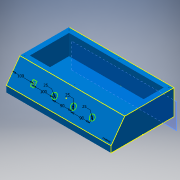
# Autodesk Inventor part: 240710_part2
Saved by Autodesk Inventor 2016 (Build 200138000, 138)
## iProperties
Created: 2024-07-10
Part Number: 240710_part2
Material: 일반
Document SubType Name: Modeling
Designer: pc
Density: 1 g/cm^3
Appearance: 기본값(1)
Author: pc
Autodesk Inventor part; units mm, degrees
ref_plane "YZ Plane" through (0, 0, 0) normal (1, 0, 0) x (0, 1, 0)
ref_plane "XZ Plane" through (0, 0, 0) normal (0, 1, 0) x (-1, 0, 0)
ref_plane "XY Plane" through (0, 0, 0) normal (0, 0, 1) x (1, 0, 0)
sketch "스케치1" plane through (0, 0, 0) normal (0, 0, 1) x (1, 0, 0)
  line L0 (250, -150) -> (-250, -150)
  line L1 (-250, -150) -> (-250, 150)
  line L2 (-250, 150) -> (250, 150)
  line L3 (250, 150) -> (250, -150)
  line L4 (250, -150) -> (-250, 150) construction
  line L5 (-250, -150) -> (250, 150) construction
  point P0 (0, 0)
  dimension "d0" = 500
  dimension "d1" = 300
  constraints: 12 end point, 2 midpoint, 2 parallel, 1 horizontal, 1 perpendicular
  measures "d0" distance of L1.end L2.end
  measures "d1" distance of L0.end L1.end
extrude "돌출1" add sketch "스케치1" along normal blind 120
sketch "스케치2" plane through (250, -150, 0) normal (1, 0, 0) x (0, 0, -1)
  line L0 (-120, 0) -> (-120, 300) projected
  line L1 (0, 0) -> (-120, 0) projected
  line L2 (-30, 0) -> (-120, 65)
  line L3 (-30, 0) -> (-30, -74.841)
  line L4 (-30, -74.841) -> (-182.9501, -91.3391)
  line L5 (-182.9501, -91.3391) -> (-221.4457, -10.4199)
  line L6 (-221.4457, -10.4199) -> (-120, 65)
  point P0 (0, 150)
  dimension "d4" = 65
  dimension "d5" = 30
  constraints: 10 end point, 2 point on line, 1 vertical
  measures "d4" distance of L2.end L0.start
  measures "d5" distance of L1.start L2.start
extrude "돌출2" cut sketch "스케치2" against normal through all contours L0 L2 L1
sketch "스케치3" plane through (0, 0, 120) normal (0, 0, 1) x (1, 0, 0)
  line L0 (-250, -85) -> (250, -85) projected
  line L1 (250, -85) -> (250, 150) projected
  line L2 (250, 150) -> (-250, 150) projected
  line L3 (-250, 150) -> (-250, -85) projected
  line L4 (-226, -61) -> (226, -61)
  line L5 (226, -61) -> (226, 126)
  line L6 (226, 126) -> (-226, 126)
  line L7 (-226, 126) -> (-226, -61)
  point P0 (0, 0)
  dimension "d8" = 24
  dimension "d9" = 24
  dimension "d10" = 24
  dimension "d11" = 24
  constraints: 8 end point, 2 parallel, 1 horizontal, 1 perpendicular
  measures "d8" distance between parallel lines of L3 L7
  measures "d9" distance between parallel lines of L2 L6
  measures "d10" distance between parallel lines of L0 L4
  measures "d11" distance between parallel lines of L1 L5
extrude "돌출3" cut sketch "스케치3" against normal blind 10 contours L7 L6 L5 L4
shell "쉘1" thickness 1.2 removed faces 5 at (-226, 63.6667, 116.6667) at (-75.3333, -61, 116.6667) at (226, 1.3333, 116.6667) at (75.3333, 126, 116.6667) at (75.3333, 1.3333, 110)
sketch "스케치4" plane through (0, 0, 120) normal (0, 0, 1) x (1, 0, 0)
  line L0 (-250, -85) -> (250, -85) projected
  line L1 (250, -85) -> (250, 150) projected
  line L2 (250, 150) -> (-250, 150) projected
  line L3 (-250, 150) -> (-250, -85) projected
  line L4 (-238, -73) -> (238, -73)
  line L5 (238, -73) -> (238, 138)
  line L6 (238, 138) -> (-238, 138)
  line L7 (-238, 138) -> (-238, -73)
  line L8 (-238, 32.5) -> (250, 32.5)
  line L9 (0, -73) -> (0, 138)
  point P0 (0, 0)
  dimension "d15" = 12
  dimension "d16" = 12
  dimension "d17" = 12
  dimension "d18" = 12
  constraints: 12 end point, 6 coincident, 4 midpoint, 2 parallel, 1 horizontal, 1 perpendicular
  measures "d15" distance between parallel lines of L0 L4
  measures "d16" distance between parallel lines of L3 L7
  measures "d17" distance between parallel lines of L2 L6
  measures "d18" distance between parallel lines of L1 L5
hole "구멍1" at (-238, -73, 120) at (-238, 138, 120) at (238, -73, 120) at (238, 138, 120) at (0, -73, 120) at (0, 138, 120) direction (0, 0, -1) diameter 4.134 depth 14.2 tip angle 118 thread size "M5x0.8" class "6H" standard "ISO Metric profile"
sketch "스케치5" plane through (-250, -150, 30) normal (0, -0.8107, 0.5855) x (1, 0, 0)
  line L0 (0, 0) -> (0, 111.018) projected
  circle A0 centre (200, 51.355) radius 12.5
  circle A1 centre (290, 51.355) radius 12.5
  circle A2 centre (380, 51.355) radius 12.5
  line L1 (109.038, 38.855) -> (90.962, 38.855)
  line L2 (90.962, 38.855) -> (90.962, 63.855)
  line L3 (90.962, 63.855) -> (109.038, 63.855)
  line L4 (109.038, 63.855) -> (109.038, 38.855)
  line L5 (109.038, 38.855) -> (90.962, 63.855) construction
  line L6 (90.962, 38.855) -> (109.038, 63.855) construction
  line L7 (455.4394, 12.1665) -> (493.5306, 12.1665) construction
  line L8 (493.5306, 12.1665) -> (493.5306, 2.974) construction
  line L9 (493.5306, 2.974) -> (455.4394, 2.974) construction
  line L10 (455.4394, 2.974) -> (455.4394, 12.1665) construction
  point P0 (250, 63.5032)
  point P1 (100, 51.355)
  dimension "d26" = 25
  dimension "d27" = 25
  dimension "d28" = 25
  dimension "d29" = 100
  dimension "d30" = 100
  dimension "d31" = 90
  dimension "d32" = 90
  constraints: 12 end point, 3 centre point, 2 midpoint, 2 parallel, 1 horizontal, 1 perpendicular, 2 other
  measures "d26" diameter of A0
  measures "d27" diameter of A1
  measures "d28" diameter of A2
  measures "d29" distance from line of L0 point (100, 51.355)
  measures "d30" distance of A0.centre point (100, 51.355)
  measures "d31" distance of A0.centre A1.centre
  measures "d32" distance of A2.centre A1.centre
sketch "스케치6" plane through (250, -150, 0) normal (1, 0, 0) x (0, 0, -1)
  line L0 (-120, 65) -> (-30, 0) projected
  line L1 (0, 0) -> (-30, 0) projected
  line L2 (0, 300) -> (0, 0) projected
  line L3 (0, 300) -> (-120, 300) projected
  line L4 (-120, 65) -> (-120, 300) projected
  point P0 (0, 150)
sketch "스케치7" plane through (250, -150, 0) normal (1, 0, 0) x (0, 0, -1)
  line L0 (-120, 65) -> (-30, 0) projected
  line L1 (0, 0) -> (-30, 0) projected
  line L2 (0, 300) -> (0, 0) projected
  line L3 (0, 300) -> (-120, 300) projected
  line L4 (-120, 65) -> (-120, 300) projected
  point P0 (0, 150)
sketch "스케치8" plane through (-250, 150, 0) normal (0, 1, 0) x (1, 0, 0)
  line L0 (0, 0) -> (500, 0) projected
  line L1 (0, 0) -> (0, -120) projected
  line L2 (500, -120) -> (0, -120) projected
  line L3 (500, 0) -> (500, -120) projected
  point P0 (250, 0)
sketch "스케치9" plane through (-250, 150, 0) normal (0, 1, 0) x (1, 0, 0)
  line L0 (446.8349, -55.3209) -> (487.5108, -55.3209) construction
  line L1 (451.514, -50.6418) -> (482.8317, -50.6418)
  line L2 (482.8317, -60) -> (451.514, -60)
  arc A0 (451.514, -50.6418) -> (451.514, -60) centre (451.514, -55.3209) ccw
  arc A1 (482.8317, -60) -> (482.8317, -50.6418) centre (482.8317, -55.3209) ccw
  line L3 (515.6985, -42.8327) -> (515.6985, 0) construction
  line L4 (432.8317, -60) -> (401.514, -60)
  line L5 (401.514, -50.6418) -> (432.8317, -50.6418)
  arc A2 (401.514, -50.6418) -> (401.514, -60) centre (401.514, -55.3209) ccw
  arc A3 (432.8317, -60) -> (432.8317, -50.6418) centre (432.8317, -55.3209) ccw
  line L6 (382.8317, -60) -> (351.514, -60)
  line L7 (351.514, -50.6418) -> (382.8317, -50.6418)
  arc A4 (351.514, -50.6418) -> (351.514, -60) centre (351.514, -55.3209) ccw
  arc A5 (382.8317, -60) -> (382.8317, -50.6418) centre (382.8317, -55.3209) ccw
  line L8 (332.8317, -60) -> (301.514, -60)
  line L9 (301.514, -50.6418) -> (332.8317, -50.6418)
  arc A6 (301.514, -50.6418) -> (301.514, -60) centre (301.514, -55.3209) ccw
  arc A7 (332.8317, -60) -> (332.8317, -50.6418) centre (332.8317, -55.3209) ccw
  line L10 (282.8317, -60) -> (251.514, -60)
  line L11 (251.514, -50.6418) -> (282.8317, -50.6418)
  arc A8 (251.514, -50.6418) -> (251.514, -60) centre (251.514, -55.3209) ccw
  arc A9 (282.8317, -60) -> (282.8317, -50.6418) centre (282.8317, -55.3209) ccw
  line L12 (232.8317, -60) -> (201.514, -60)
  line L13 (201.514, -50.6418) -> (232.8317, -50.6418)
  arc A10 (201.514, -50.6418) -> (201.514, -60) centre (201.514, -55.3209) ccw
  arc A11 (232.8317, -60) -> (232.8317, -50.6418) centre (232.8317, -55.3209) ccw
  line L14 (182.8317, -60) -> (151.514, -60)
  line L15 (151.514, -50.6418) -> (182.8317, -50.6418)
  arc A12 (151.514, -50.6418) -> (151.514, -60) centre (151.514, -55.3209) ccw
  arc A13 (182.8317, -60) -> (182.8317, -50.6418) centre (182.8317, -55.3209) ccw
  line L16 (132.8317, -60) -> (101.514, -60)
  line L17 (101.514, -50.6418) -> (132.8317, -50.6418)
  arc A14 (101.514, -50.6418) -> (101.514, -60) centre (101.514, -55.3209) ccw
  arc A15 (132.8317, -60) -> (132.8317, -50.6418) centre (132.8317, -55.3209) ccw
  line L18 (82.8317, -60) -> (51.514, -60)
  line L19 (51.514, -50.6418) -> (82.8317, -50.6418)
  arc A16 (51.514, -50.6418) -> (51.514, -60) centre (51.514, -55.3209) ccw
  arc A17 (82.8317, -60) -> (82.8317, -50.6418) centre (82.8317, -55.3209) ccw
  line L20 (482.8317, -45) -> (451.514, -45)
  line L21 (451.514, -35.6418) -> (482.8317, -35.6418)
  arc A18 (451.514, -35.6418) -> (451.514, -45) centre (451.514, -40.3209) ccw
  arc A19 (482.8317, -45) -> (482.8317, -35.6418) centre (482.8317, -40.3209) ccw
  line L22 (432.8317, -45) -> (401.514, -45)
  line L23 (401.514, -35.6418) -> (432.8317, -35.6418)
  arc A20 (401.514, -35.6418) -> (401.514, -45) centre (401.514, -40.3209) ccw
  arc A21 (432.8317, -45) -> (432.8317, -35.6418) centre (432.8317, -40.3209) ccw
  line L24 (382.8317, -45) -> (351.514, -45)
  line L25 (351.514, -35.6418) -> (382.8317, -35.6418)
  arc A22 (351.514, -35.6418) -> (351.514, -45) centre (351.514, -40.3209) ccw
  arc A23 (382.8317, -45) -> (382.8317, -35.6418) centre (382.8317, -40.3209) ccw
  line L26 (332.8317, -45) -> (301.514, -45)
  line L27 (301.514, -35.6418) -> (332.8317, -35.6418)
  arc A24 (301.514, -35.6418) -> (301.514, -45) centre (301.514, -40.3209) ccw
  arc A25 (332.8317, -45) -> (332.8317, -35.6418) centre (332.8317, -40.3209) ccw
  line L28 (282.8317, -45) -> (251.514, -45)
  line L29 (251.514, -35.6418) -> (282.8317, -35.6418)
  arc A26 (251.514, -35.6418) -> (251.514, -45) centre (251.514, -40.3209) ccw
  arc A27 (282.8317, -45) -> (282.8317, -35.6418) centre (282.8317, -40.3209) ccw
  line L30 (232.8317, -45) -> (201.514, -45)
  line L31 (201.514, -35.6418) -> (232.8317, -35.6418)
  arc A28 (201.514, -35.6418) -> (201.514, -45) centre (201.514, -40.3209) ccw
  arc A29 (232.8317, -45) -> (232.8317, -35.6418) centre (232.8317, -40.3209) ccw
  line L32 (182.8317, -45) -> (151.514, -45)
  line L33 (151.514, -35.6418) -> (182.8317, -35.6418)
  arc A30 (151.514, -35.6418) -> (151.514, -45) centre (151.514, -40.3209) ccw
  arc A31 (182.8317, -45) -> (182.8317, -35.6418) centre (182.8317, -40.3209) ccw
  line L34 (132.8317, -45) -> (101.514, -45)
  line L35 (101.514, -35.6418) -> (132.8317, -35.6418)
  arc A32 (101.514, -35.6418) -> (101.514, -45) centre (101.514, -40.3209) ccw
  arc A33 (132.8317, -45) -> (132.8317, -35.6418) centre (132.8317, -40.3209) ccw
  line L36 (82.8317, -45) -> (51.514, -45)
  line L37 (51.514, -35.6418) -> (82.8317, -35.6418)
  arc A34 (51.514, -35.6418) -> (51.514, -45) centre (51.514, -40.3209) ccw
  arc A35 (82.8317, -45) -> (82.8317, -35.6418) centre (82.8317, -40.3209) ccw
  line L38 (482.8317, -30) -> (451.514, -30)
  line L39 (451.514, -20.6418) -> (482.8317, -20.6418)
  arc A36 (451.514, -20.6418) -> (451.514, -30) centre (451.514, -25.3209) ccw
  arc A37 (482.8317, -30) -> (482.8317, -20.6418) centre (482.8317, -25.3209) ccw
  line L40 (432.8317, -30) -> (401.514, -30)
  line L41 (401.514, -20.6418) -> (432.8317, -20.6418)
  arc A38 (401.514, -20.6418) -> (401.514, -30) centre (401.514, -25.3209) ccw
  arc A39 (432.8317, -30) -> (432.8317, -20.6418) centre (432.8317, -25.3209) ccw
  line L42 (382.8317, -30) -> (351.514, -30)
  line L43 (351.514, -20.6418) -> (382.8317, -20.6418)
  arc A40 (351.514, -20.6418) -> (351.514, -30) centre (351.514, -25.3209) ccw
  arc A41 (382.8317, -30) -> (382.8317, -20.6418) centre (382.8317, -25.3209) ccw
  line L44 (332.8317, -30) -> (301.514, -30)
  line L45 (301.514, -20.6418) -> (332.8317, -20.6418)
  arc A42 (301.514, -20.6418) -> (301.514, -30) centre (301.514, -25.3209) ccw
  arc A43 (332.8317, -30) -> (332.8317, -20.6418) centre (332.8317, -25.3209) ccw
  line L46 (282.8317, -30) -> (251.514, -30)
  line L47 (251.514, -20.6418) -> (282.8317, -20.6418)
  arc A44 (251.514, -20.6418) -> (251.514, -30) centre (251.514, -25.3209) ccw
  arc A45 (282.8317, -30) -> (282.8317, -20.6418) centre (282.8317, -25.3209) ccw
  line L48 (232.8317, -30) -> (201.514, -30)
  line L49 (201.514, -20.6418) -> (232.8317, -20.6418)
  arc A46 (201.514, -20.6418) -> (201.514, -30) centre (201.514, -25.3209) ccw
  arc A47 (232.8317, -30) -> (232.8317, -20.6418) centre (232.8317, -25.3209) ccw
  line L50 (182.8317, -30) -> (151.514, -30)
  line L51 (151.514, -20.6418) -> (182.8317, -20.6418)
  arc A48 (151.514, -20.6418) -> (151.514, -30) centre (151.514, -25.3209) ccw
  arc A49 (182.8317, -30) -> (182.8317, -20.6418) centre (182.8317, -25.3209) ccw
  line L52 (132.8317, -30) -> (101.514, -30)
  line L53 (101.514, -20.6418) -> (132.8317, -20.6418)
  arc A50 (101.514, -20.6418) -> (101.514, -30) centre (101.514, -25.3209) ccw
  arc A51 (132.8317, -30) -> (132.8317, -20.6418) centre (132.8317, -25.3209) ccw
  line L54 (82.8317, -30) -> (51.514, -30)
  line L55 (51.514, -20.6418) -> (82.8317, -20.6418)
  arc A52 (51.514, -20.6418) -> (51.514, -30) centre (51.514, -25.3209) ccw
  arc A53 (82.8317, -30) -> (82.8317, -20.6418) centre (82.8317, -25.3209) ccw
  point P0 (250, 0)
  point P1 (467.1729, -55.3209)
  dimension "d35" = 50
  dimension "d38" = 15
  constraints: 114 end point, 110 point on circle, 54 centre point, 4 tangent, 2 horizontal, 2 point on line, 2 vertical, 1 collinear, 1 midpoint, 1 parallel, 259 other
  measures "d35" distance of L2.start L4.start
  measures "d38" distance of L2.start L20.start
extrude "돌출4" cut sketch "스케치9" against normal blind 10
extrude "돌출5" cut sketch "스케치5" against normal blind 10
